Autodesk Inventor part; units mm, degrees
(part 2 of 2)
hole "Tapping 9" at (-51.0307, -19.2083, 7.5) direction (-0.0241419, 0.9997085, 0) diameter 4 depth 10 tip angle 118
hole "Tapping 10" at (22.2132, -15.6289, 7.5) direction (-0.073682, 0.9972818, 0) diameter 4 depth 10 tip angle 118
extrude "Extrusion6" cut sketch "Sketch5" against normal blind 35.7 contours A2 | A3
sketch "Sketch10" plane through (0, 0, 15) normal (0, 0, 1) x (1, 0, 0)
  circle A0 centre (-41.0917, 17.7797) radius 1.6
  circle A1 centre (-22.0917, 17.7797) radius 1.6
  circle A2 centre (-47.8417, -12.9703) radius 1.6
  circle A3 centre (-15.3417, -12.9703) radius 1.6
  circle A4 centre (-80.5289, 0.8706) radius 13.2395 construction
  arc A5 (-87.8309, -10.1732) -> (-72.9926, -10.0147) centre (-80.5289, 0.8706) ccw projected
  point P0 (0, 0)
  point P1 (0.0492, 0.0183)
  dimension "d217" = 32.5
  dimension "d218" = 30.75
  dimension "d219" = 19
  dimension "d220" = 6.75
  dimension "d221" = 32.6872
  dimension "d222" = 13.8408
  constraints: 5 centre point, 2 coincident, 2 horizontal alignment
  measures "d217" distance of A3.centre A2.centre
  measures "d218" vertical distance of A1.centre A3.centre
  measures "d219" distance of A0.centre A1.centre
  measures "d220" horizontal distance of A3.centre A1.centre
  measures "d221" horizontal distance of A2.centre A4.centre
  measures "d222" vertical distance of A2.centre A4.centre
extrude "Extrusion8" cut sketch "Sketch10" against normal blind 10
body "Solid3"
